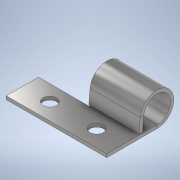
# Autodesk Inventor part: dobradica
Saved by Autodesk Inventor 2022 (Build 260153000, 153)
## iProperties
Created: 2022-02-18
Part Number: dobradica
Material: Ferro, maleável
Document SubType Name: Modelagem
Designer: mathe
Density: 7.15 g/cm^3
Appearance: Semipolido
Author: mathe
Autodesk Inventor part; units mm, degrees
ref_plane "YZ Plane" through (0, 0, 0) normal (1, 0, 0) x (0, 1, 0)
ref_plane "XZ Plane" through (0, 0, 0) normal (0, 1, 0) x (-1, 0, 0)
ref_plane "XY Plane" through (0, 0, 0) normal (0, 0, 1) x (1, 0, 0)
sketch "Esboço1" plane through (0, 0, 0) normal (0, 0, 1) x (1, 0, 0)
  line L0 (0, 0) -> (15, 0)
  dimension "d0" = 15
  measures "d0" distance of L0.start L0.end
contour flange "Flange de contorno1" sketch "Esboço1" thickness 0.5 bend radius 0.5 width 10 along (0, 0, 1) mid plane no both sides no wall seen from (7.5, 0, 0) lies toward (0, -1, 0) curves L0
bend "Vergadura1"
corner "Canto1"
sketch "Esboço2" plane through (0, 0, 10) normal (0, 1, 0) x (1, 0, 0)
  line L0 (0, 10) -> (15, 10) projected
  line L1 (0, 10) -> (7.5, 10)
  line L2 (7.5, 10) -> (7.5, 5)
  line L3 (7.5, 5) -> (0, 5)
  line L4 (0, 5) -> (0, 10)
  dimension "d12" = 5
  constraints: 8 end point, 2 parallel, 1 horizontal, 1 perpendicular
  measures "d12" distance of L1.end L2.end
extrude "Recortar1" cut sketch "Esboço2" against normal blind 0.5
sketch "Esboço3" plane through (15, 0, 2.5) normal (1, 0, 0) x (0, 1, 0)
  line L0 (-0.5, 0) -> (0, 0)
  arc A0 (0, 0) -> (2.1743, 1.9924) centre (2, 0) ccw
  line L1 (2.1743, 1.9924) -> (0.125, 2.1717)
  line L2 (0.125, 2.1717) -> (0.1686, 2.6698)
  line L3 (0.1686, 2.6698) -> (2.2179, 2.4905)
  arc A1 (-0.5, 0) -> (2.2179, 2.4905) centre (2, 0) ccw
  constraints: 8 end point, 4 point on circle
hem "Borda1" sketch "Esboço3" thickness 0.5 along (-1, 0, 0) edges at (11.25, 0, 0)
sketch "Esboço4" plane through (0, 0, 10) normal (0, 1, 0) x (1, 0, 0)
  point P0 (0, 10)
  point P1 (4, 2.5)
  point P2 (11, 2.5)
hole "Furo1" at (4, 0, 7.5) at (11, 0, 7.5) direction (0, -1, 0) diameter 2 end through all
sketch "Esboço5" plane through (0, 0, 10) normal (0, 1, 0) x (1, 0, 0)
  line L0 (0, 5) -> (0, 0) projected
  line L1 (7.5, 4.8302) -> (7.5, 5.3283) projected
  line L2 (0, 5) -> (7.5, 5)
  line L3 (7.5, 5) -> (7.5, 4.8302)
  line L4 (7.5, 4.8302) -> (0, 4.8302)
  line L5 (0, 4.8302) -> (0, 5)
  point P0 (0, 10)
  constraints: 8 end point, 2 parallel, 1 horizontal, 1 perpendicular
extrude "Recortar2" cut sketch "Esboço5" against normal blind 0.5
equation "\"d13\" = Espessura"
equation "\"d1\" = Espessura"
equation "\"d15\" = Largura_alívio_de_vergadura"
equation "\"d16\" = Profundidade_alívio_de_vergadura"
equation "\"d17\" = Remanescente_mínimo"
equation "\"d18\" = Raiodetransição"
equation "\"d21\" = d20"
equation "\"d27\" = Espessura"
equation "\"d29\" = Espessura"
equation "\"d2\" = Largura_alívio_de_vergadura"
equation "\"d3\" = Profundidade_alívio_de_vergadura"
equation "\"d4\" = Remanescente_mínimo"
equation "\"d5\" = Raiodetransição"
equation "\"d7\" = Raio_vergadura"
equation "\"d9\" = Tamanho_alívio_de_dobra"
equation "\"d10\" = TamanhoFolga"
equation "\"d11\" = Tamanho_de_raio_de_Jacobi"
equation "\"Raio_vergadura\" = Espessura"
equation "\"Largura_alívio_de_vergadura\" = Espessura"
equation "\"Profundidade_alívio_de_vergadura\" = 0.5 * Espessura"
equation "\"Tamanho_alívio_de_dobra\" = 4 * Espessura"
equation "\"Remanescente_mínimo\" = 2 * Espessura"
equation "\"Raiodetransição\" = Raio_vergadura"
equation "\"Tamanho_de_raio_de_Jacobi\" = Raio_vergadura"
equation "\"TamanhoFolga\" = Espessura"
equation "\"Espessura\" = 0.5"
equation "\"d20\" = 2"
